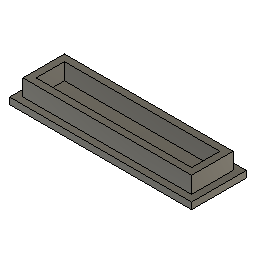
openepaper_diy_ap_dekseltje v1 (Autodesk Fusion 360 design; units mm, degrees)
Autodesk Fusion 360 part; units mm, degrees
sketch "Sketch1" plane through (0, 0, 0) normal (0, 0, 1) x (1, 0, 0)
  line L0 (0, 0) -> (32.9, 0)
  line L1 (32.9, 0) -> (32.9, 9.9)
  line L2 (32.9, 9.9) -> (0, 9.9)
  line L3 (0, 9.9) -> (0, 0)
  dimension "d1" = 32.9
  dimension "d2" = 9.9
  constraint horizontal L0
  constraint vertical L1
  constraint horizontal L2
  constraint vertical L3
  constraint coincident L0.start L3.end
  measures "d1" distance of L0.start L0.end
  measures "d2" distance of L0.start L2.end
extrude "Extrude1" add sketch "Sketch1" along normal blind 1.2
sketch "Sketch2" plane through (0, 0, 1.2) normal (0, 0, 1) x (-1, 0, 0)
  line L0 (0, -9.9) -> (0, 0)
  line L1 (0, 0) -> (-32.9, 0)
  line L2 (-32.9, 0) -> (-32.9, -9.9)
  line L3 (-32.9, -9.9) -> (0, -9.9)
  line L4 (-1.2, -8.7) -> (-31.7, -8.7)
  line L5 (-31.7, -8.7) -> (-31.7, -1.2)
  line L6 (-31.7, -1.2) -> (-1.2, -1.2)
  line L7 (-1.2, -1.2) -> (-1.2, -8.7)
  line L8 (-2.4, -7.5) -> (-30.5, -7.5)
  line L9 (-30.5, -7.5) -> (-30.5, -2.4)
  line L10 (-30.5, -2.4) -> (-2.4, -2.4)
  line L11 (-2.4, -2.4) -> (-2.4, -7.5)
  dimension "d5" = 1.2
  dimension "d6" = 1.2
  dimension "d7" = 1.2
  dimension "d8" = 1.2
  dimension "d9" = 1.2
  dimension "d10" = 1.2
  dimension "d11" = 1.2
  dimension "d12" = 1.2
  constraint horizontal L4
  constraint vertical L5
  constraint horizontal L6
  constraint vertical L7
  constraint horizontal L8
  constraint vertical L9
  constraint horizontal L10
  constraint vertical L11
  measures "d5" distance of L2 L5
  measures "d6" distance of L1 L6
  measures "d7" distance of L3 L4
  measures "d8" distance of L0 L7
  measures "d9" distance of L5 L9
  measures "d10" distance of L6 L10
  measures "d11" distance of L7 L11
  measures "d12" distance of L4 L8
extrude "Extrude2" add sketch "Sketch2" along normal blind 3 contours L4 L5 L6 L7
equation "d7 = d5"
equation "d8 = d6"
equation "d9 = d5"
equation "d10 = d6"
equation "d11 = d8"
equation "d12 = d7"
